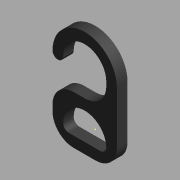
# Autodesk Inventor part: Part2
Saved by Autodesk Inventor 2019.3 (Build 233278000, 278)
## iProperties
Part Number: Part2
Material: Generic
Document SubType Name: Modeling
Designer: Frienddo
Appearance: Default
Author: Frienddo
Autodesk Inventor part; units mm, degrees
ref_plane "YZ Plane" through (0, 0, 0) normal (1, 0, 0) x (0, 1, 0)
ref_plane "XZ Plane" through (0, 0, 0) normal (0, 1, 0) x (-1, 0, 0)
ref_plane "XY Plane" through (0, 0, 0) normal (0, 0, 1) x (1, 0, 0)
sketch "Sketch1" plane through (0, 0, 0) normal (0, 0, 1) x (1, 0, 0)
  point P0 (0, 0)
sketch "Sketch2" plane through (0, 0, 0) normal (0, 0, 1) x (1, 0, 0)
  arc A0 (20, 0) -> (-20, 0) centre (0, 0) ccw
  line L0 (-15, -5) -> (15, -5)
  arc A1 (-20, 0) -> (-15, -5) centre (-15, 0) ccw
  arc A2 (15, -5) -> (20, 0) centre (15, 0) ccw
  line L1 (-48.289, 0) -> (48.289, 0) projected
  arc A3 (20.35, 0) -> (-20.35, 0) centre (0, 0) ccw
  arc A4 (15, -5.35) -> (20.35, 0) centre (15, 0) ccw
  line L2 (15, -5.35) -> (-15, -5.35)
  arc A5 (-20.35, 0) -> (-15, -5.35) centre (-15, 0) ccw
  line L3 (-10.35, -15.35) -> (10.35, -15.35)
  line L4 (30.35, 4.65) -> (30.35, 54.3)
  arc A6 (30.35, 54.3) -> (-30.35, 54.3125) centre (0, 54.3) ccw
  arc A7 (20.35, 54.3104) -> (-20.35, 54.3084) centre (0, 54.3) ccw
  line L5 (20.35, 54.3104) -> (20.35, 50.35)
  line L6 (0.35, 30.35) -> (-10.35, 30.35)
  line L7 (-30.35, 10.35) -> (-30.35, 4.65)
  arc A8 (-10.35, 30.35) -> (-30.35, 10.35) centre (-10.35, 10.35) ccw
  arc A9 (0.35, 30.35) -> (20.35, 50.35) centre (0.35, 50.35) ccw
  arc A10 (-30.35, 4.65) -> (-10.35, -15.35) centre (-10.35, 4.65) ccw
  arc A11 (10.35, -15.35) -> (30.35, 4.65) centre (10.35, 4.65) ccw
  arc A12 (-30.35, 54.3125) -> (-20.35, 54.3084) centre (-25.35, 54.3104) ccw
  point P0 (0, 20.35)
  point P1 (0.0062, 84.65)
  dimension "d0" = 5
  dimension "d1" = 20
  dimension "d2" = 5
  dimension "d3" = 0.35
  dimension "d4" = 10
  dimension "d5" = 10
  dimension "d6" = 10
  dimension "d7" = 10
  dimension "d8" = 10
  dimension "d9" = 10
  dimension "d11" = 100
  dimension "d12" = 20
  constraints: 28 point on circle, 14 end point, 13 centre point, 13 tangent, 4 coincident, 4 equal radius, 3 horizontal, 3 perpendicular, 2 horizontal alignment, 2 point on line, 9 other
  measures "d0" radius of A1
  measures "d1" radius of A0
  measures "d2" distance from line of A0.end L0
  measures "d3" radial gap between concentric circles of A0 A3
  measures "d4" distance from line of L7 A3.end
  measures "d5" distance from line of L4 A3.start
  measures "d6" distance between parallel lines of L3 L2
  measures "d7" distance from line of L6 point (0, 20.35)
  measures "d8" distance between parallel lines of L4 L5
  measures "d9" radial gap between concentric circles of A6 A7
  measures "d11" distance from line of L3 point (0.006, 84.65)
  measures "d12" radius of A8
extrude "Extrusion1" add sketch "Sketch2" along normal blind 10 contours A3 L1 A10 L7 A8 L6 A9 L5 A7 A12 A6 L4 A11 | L1 A11 L3 A10 A5 L2 A4
body "Solid1"
